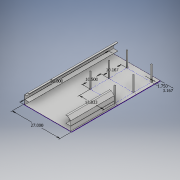
# Autodesk Inventor part: ROOM_B164
Saved by Autodesk Inventor 2019 (Build 230136000, 136)
## iProperties
Created: 2020-10-30
Part Number: ROOM_B164
Material: Generic
Document SubType Name: Modeling
Designer: close
Density: 1 g/cm^3
Appearance: Default
Author: close
Autodesk Inventor part; units mm, degrees
ref_plane "YZ Plane" through (0, 0, 0) normal (1, 0, 0) x (0, 1, 0)
ref_plane "XZ Plane" through (0, 0, 0) normal (0, 1, 0) x (-1, 0, 0)
ref_plane "XY Plane" through (0, 0, 0) normal (0, 0, 1) x (1, 0, 0)
sketch "Sketch1" plane through (0, 0, 0) normal (0, 1, 0) x (-1, 0, 0)
  line L0 (0, 0) -> (8229.6, 0)
  line L1 (8229.6, 0) -> (8229.6, -15240)
  line L2 (8229.6, -15240) -> (0, -15240)
  line L3 (0, -15240) -> (0, 0)
  line L4 (533.4, -7975.6) -> (533.4, -11176) construction
  line L5 (533.4, -11176) -> (533.4, -14274.8) construction
  line L6 (4749.8, -7975.6) -> (4749.8, -11176) construction
  line L7 (4749.8, -11176) -> (4749.8, -14274.8) construction
  line L8 (4749.8, -14274.8) -> (533.4, -14274.8) construction
  line L9 (4749.8, -7975.6) -> (533.4, -7975.6) construction
  line L10 (533.4, -11176) -> (4749.8, -11176) construction
  dimension "d0" = 15240
  dimension "d1" = 8229.6
  dimension "d2" = 3200.4
  dimension "d3" = 3098.8
  dimension "d4" = 4216.4
  dimension "d5" = 533.4
  dimension "d6" = 965.2
  constraints: 22 end point, 4 parallel, 2 collinear, 2 horizontal, 2 perpendicular, 1 coincident, 1 vertical
  measures "d0" distance of L0.end L1.end
  measures "d1" distance of L0.start L0.end
  measures "d2" distance of L6.start L6.end
  measures "d3" distance of L6.end L7.end
  measures "d4" distance of L6.start L4.start
  measures "d5" distance from line of L5.end L3
  measures "d6" distance from line of L2 L5.end
extrude "Extrusion1" add sketch "Sketch1" along normal blind 25.4
sketch "Sketch2" plane through (0, 25.4, 0) normal (0, 1, 0) x (1, 0, 0)
  line L0 (-4673.6, 8051.8) -> (-4826, 8051.8)
  line L1 (-4826, 8051.8) -> (-4826, 7899.4)
  line L2 (-4826, 7899.4) -> (-4673.6, 7899.4)
  line L3 (-4673.6, 7899.4) -> (-4673.6, 8051.8)
  line L4 (-4673.6, 8051.8) -> (-4826, 7899.4) construction
  line L5 (-4826, 8051.8) -> (-4673.6, 7899.4) construction
  line L6 (-457.2, 7899.4) -> (-609.6, 7899.4)
  line L7 (-609.6, 7899.4) -> (-609.6, 8051.8)
  line L8 (-609.6, 8051.8) -> (-457.2, 8051.8)
  line L9 (-457.2, 8051.8) -> (-457.2, 7899.4)
  line L10 (-457.2, 7899.4) -> (-609.6, 8051.8) construction
  line L11 (-609.6, 7899.4) -> (-457.2, 8051.8) construction
  line L12 (-4673.6, 11099.8) -> (-4826, 11099.8)
  line L13 (-4826, 11099.8) -> (-4826, 11252.2)
  line L14 (-4826, 11252.2) -> (-4673.6, 11252.2)
  line L15 (-4673.6, 11252.2) -> (-4673.6, 11099.8)
  line L16 (-4673.6, 11099.8) -> (-4826, 11252.2) construction
  line L17 (-4826, 11099.8) -> (-4673.6, 11252.2) construction
  line L18 (-457.2, 11099.8) -> (-609.6, 11099.8)
  line L19 (-609.6, 11099.8) -> (-609.6, 11252.2)
  line L20 (-609.6, 11252.2) -> (-457.2, 11252.2)
  line L21 (-457.2, 11252.2) -> (-457.2, 11099.8)
  line L22 (-457.2, 11099.8) -> (-609.6, 11252.2) construction
  line L23 (-609.6, 11099.8) -> (-457.2, 11252.2) construction
  line L24 (-457.2, 14198.6) -> (-609.6, 14198.6)
  line L25 (-609.6, 14198.6) -> (-609.6, 14351)
  line L26 (-609.6, 14351) -> (-457.2, 14351)
  line L27 (-457.2, 14351) -> (-457.2, 14198.6)
  line L28 (-457.2, 14198.6) -> (-609.6, 14351) construction
  line L29 (-609.6, 14198.6) -> (-457.2, 14351) construction
  line L30 (-4673.6, 14198.6) -> (-4826, 14198.6)
  line L31 (-4826, 14198.6) -> (-4826, 14351)
  line L32 (-4826, 14351) -> (-4673.6, 14351)
  line L33 (-4673.6, 14351) -> (-4673.6, 14198.6)
  line L34 (-4673.6, 14198.6) -> (-4826, 14351) construction
  line L35 (-4826, 14198.6) -> (-4673.6, 14351) construction
  point P0 (0, 0)
  point P1 (-4749.8, 14274.8)
  point P2 (-533.4, 14274.8)
  point P3 (-533.4, 11176)
  point P4 (-4749.8, 11176)
  point P5 (-4749.8, 7975.6)
  point P6 (-533.4, 7975.6)
  dimension "d9" = 152.4
  dimension "d10" = 152.4
  dimension "d11" = 152.4
  dimension "d12" = 152.4
  dimension "d13" = 152.4
  dimension "d14" = 152.4
  dimension "d15" = 152.4
  dimension "d16" = 152.4
  dimension "d17" = 152.4
  dimension "d18" = 152.4
  dimension "d19" = 152.4
  constraints: 72 end point, 12 midpoint, 12 parallel, 6 horizontal, 6 perpendicular, 1 point on line
  measures "d9" distance of L0.end L1.end
  measures "d10" distance of L0.start L0.end
  measures "d11" distance of L12.start L12.end
  measures "d12" distance of L12.end L13.end
  measures "d13" distance of L30.start L30.end
  measures "d14" distance of L30.end L31.end
  measures "d15" distance of L6.end L7.end
  measures "d16" distance of L6.start L6.end
  measures "d17" distance of L18.end L19.end
  measures "d18" distance of L18.start L18.end
  measures "d19" distance of L24.end L25.end
extrude "Extrusion2" add sketch "Sketch2" along normal blind 2641.6
sketch "Sketch3" plane through (0, 25.4, 0) normal (0, 1, 0) x (1, 0, 0)
  line L0 (-8229.6, 0) -> (-7264.4, 0)
  line L1 (-7264.4, 0) -> (-7264.4, 15240)
  line L2 (-7264.4, 15240) -> (-8229.6, 15240)
  line L3 (-8229.6, 15240) -> (-8229.6, 0)
  line L4 (0, 7493) -> (-965.2, 7493)
  line L5 (-965.2, 7493) -> (-965.2, 0)
  line L6 (-965.2, 0) -> (0, 0)
  line L7 (0, 0) -> (0, 7493)
  line L8 (-8229.6, 15240) -> (-8229.6, 0) projected
  line L9 (0, 15240) -> (-8229.6, 15240) projected
  line L10 (-8229.6, 0) -> (0, 0) projected
  line L11 (0, 0) -> (0, 15240) projected
  line L12 (-609.6, 7899.4) -> (-457.2, 7899.4) projected
  dimension "d22" = 965.2
  dimension "d23" = 0
  dimension "d24" = 0
  dimension "d25" = 0
  dimension "d26" = 965.2
  dimension "d27" = 0
  dimension "d28" = 406.4
  dimension "d29" = 0
  constraints: 16 end point, 4 parallel, 2 horizontal, 2 perpendicular
  measures "d22" distance between parallel lines of L3 L1
  measures "d23" distance between parallel lines of L8 L3
  measures "d24" distance between parallel lines of L9 L2
  measures "d25" distance between parallel lines of L10 L0
  measures "d26" distance between parallel lines of L7 L5
  measures "d27" distance between parallel lines of L11 L7
  measures "d28" distance between parallel lines of L12 L4
  measures "d29" distance between parallel lines of L10 L6
extrude "Extrusion3" add sketch "Sketch3" along normal blind 2032 contours L3 L2 L1 L0 | L5 L4 L7 L6
sketch "Sketch4" plane through (-8229.6, 0, 0) normal (0, 0, 1) x (1, 0, 0)
  line L0 (685.8, 2057.4) -> (165.1, 1524)
  line L1 (165.1, 1524) -> (165.1, 774.7)
  line L2 (0, 0) -> (0, 2057.4) projected
  line L3 (165.1, 774.7) -> (152.4, 774.7)
  line L4 (152.4, 774.7) -> (152.4, 800.1)
  line L5 (152.4, 800.1) -> (165.1, 800.1)
  line L6 (165.1, 800.1) -> (165.1, 0)
  line L7 (8229.6, 0) -> (0, 0) projected
  line L8 (965.2, 25.4) -> (965.2, 2057.4) projected
  line L9 (965.2, 2006.6) -> (671.7055, 2006.6)
  line L10 (671.7055, 2006.6) -> (200.596, 1524)
  line L11 (200.596, 1524) -> (508, 1524)
  line L12 (508, 1524) -> (508, 1498.6)
  line L13 (508, 1498.6) -> (203.2, 1498.6)
  line L14 (203.2, 1498.6) -> (203.2, 774.7)
  line L15 (203.2, 774.7) -> (965.2, 774.7)
  line L16 (965.2, 800.1) -> (203.2, 800.1)
  line L17 (203.2, 0) -> (203.2, 800.1)
  line L18 (165.1, 0) -> (203.2, 0)
  line L19 (0, 2057.4) -> (965.2, 2057.4) projected
  line L20 (685.8, 2057.4) -> (965.2, 2057.4)
  line L21 (965.2, 25.4) -> (7264.4, 25.4) projected
  line L22 (965.2, 25.4) -> (203.2, 25.4)
  line L23 (8229.6, 0) -> (8229.6, 2057.4) projected
  line L24 (4114.8, 3713.7575) -> (4114.8, -1399.6684) construction
  line L25 (8229.6, 2057.4) -> (7264.4, 2057.4) projected
  line L26 (7264.4, 2057.4) -> (7543.8, 2057.4)
  line L27 (7543.8, 2057.4) -> (8077.2, 1579.9552)
  line L28 (8077.2, 1579.9552) -> (8077.2, 800.1)
  line L29 (8077.2, 800.1) -> (8102.6, 800.1)
  line L30 (8102.6, 800.1) -> (8102.6, 774.7)
  line L31 (8102.6, 774.7) -> (8077.2, 774.7)
  line L32 (8077.2, 774.7) -> (8077.2, 0)
  line L33 (7264.4, 25.4) -> (7264.4, 2057.4) projected
  line L34 (7264.4, 2057.4) -> (7264.4, 2006.6)
  line L35 (7264.4, 2006.6) -> (7541.0175, 2006.6)
  line L36 (7541.0175, 2006.6) -> (8051.8, 1549.4)
  line L37 (8051.8, 1549.4) -> (7747, 1549.4)
  line L38 (7747, 1549.4) -> (7747, 1524)
  line L39 (7747, 1524) -> (8051.8, 1524)
  line L40 (8051.8, 1524) -> (8051.8, 800.1)
  line L41 (8051.8, 800.1) -> (7264.4, 800.1)
  line L42 (7264.4, 774.7) -> (8051.8, 774.7)
  line L43 (8051.8, 774.7) -> (8051.8, 0)
  line L44 (8051.8, 0) -> (8077.2, 0)
  line L45 (0, 0) -> (8229.6, 0) projected
  line L46 (7264.4, 800.1) -> (7264.4, 774.7)
  line L47 (7264.4, 25.4) -> (8229.6, 25.4) projected
  line L48 (7264.4, 25.4) -> (8051.8, 25.4)
  line L49 (8077.2, 25.4) -> (8229.6, 25.4)
  point P0 (7620, 25.4)
  dimension "d33" = 279.4
  dimension "d34" = 152.4
  dimension "d35" = 38.1
  dimension "d36" = 25.4
  dimension "d37" = 304.8
  dimension "d38" = 25.4
  dimension "d40" = 723.9
  dimension "d41" = 25.4
  dimension "d42" = 749.3
  dimension "d43" = 12.7
  dimension "d44" = 0
  dimension "d47" = 8229.6
  dimension "d48" = 4114.8
  dimension "d49" = 50.8
  dimension "d50" = 50.8
  dimension "d51" = 279.4
  dimension "d53" = 25.4
  dimension "d55" = 25.4
  dimension "d56" = 749.3
  dimension "d57" = 723.9
  dimension "d61" = 25.4
  dimension "d62" = 0
  dimension "d65" = 304.8
  dimension "d66" = 152.4
  dimension "d67" = 25.4
  dimension "d68" = 25.4
  dimension "d69" = 0
  constraints: 80 end point, 28 point on line, 17 perpendicular, 6 parallel, 4 collinear, 2 horizontal, 1 coincident, 1 vertical
  measures "d33" distance of L8.end L0.start
  measures "d34" distance between parallel lines of L2 L4
  measures "d35" distance between parallel lines of L1 L14
  measures "d36" distance between parallel lines of L11 L13
  measures "d37" distance of L12.end L13.end
  measures "d38" distance between parallel lines of L0 L10
  measures "d40" distance between parallel lines of L15 L13
  measures "d41" distance between parallel lines of L15 L16
  measures "d42" distance from line of L8.start L15
  measures "d43" distance from line of L4.end L1
  measures "d44" distance from line of L11 L0.end
  measures "d47" distance between parallel lines of L23 L2
  measures "d48" distance between parallel lines of L23 L24
  measures "d49" distance between parallel lines of L19 L9
  measures "d50" distance between parallel lines of L25 L35
  measures "d51" distance of L25.end L26.end
  measures "d53" distance between parallel lines of L39 L37
  measures "d55" distance between parallel lines of L42 L41
  measures "d56" distance between parallel lines of L21 L42
  measures "d57" distance between parallel lines of L41 L39
  measures "d61" distance between parallel lines of L31 L29
  measures "d62" horizontal distance of L39.end L36.end
  measures "d65" distance of L36.end L37.end
  measures "d66" distance between parallel lines of L23 L28
  measures "d67" distance between parallel lines of L28 L30
  measures "d68" distance between parallel lines of L28 L40
  measures "d69" distance from line of L42 L31.end
extrude "Extrusion4" cut sketch "Sketch4" against normal up to surface (15240 mm away) contours L0 L1 L5 L4 L3 L6 L7 L2 L19 | L8 L16 L14 L13 L12 L11 L10 L9 | L8 L22 L17 L15
extrude "Extrusion5" cut sketch "Sketch4" against normal up to surface (7493 mm away) contours L47 L33 L42 L43 | L32 L31 L30 L29 L28 L27 L25 L23 L47 | L33 L35 L36 L37 L38 L39 L40 L41
equation "\"d10\" = d9"
equation "\"d11\" = d10"
equation "\"d12\" = d11"
equation "\"d13\" = d11"
equation "\"d14\" = d12"
equation "\"d15\" = d10"
equation "\"d16\" = d10"
equation "\"d17\" = d15"
equation "\"d18\" = d17"
equation "\"d19\" = d17"
equation "\"d48\" = 0.5 * d47"
equation "\"d50\" = d49"
equation "\"d51\" = d33"
equation "\"d53\" = d36"
equation "\"d55\" = d41"
equation "\"d56\" = d42"
equation "\"d57\" = d40"
equation "\"d61\" = d55"
body "Solid1"
